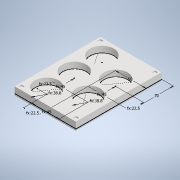
# Autodesk Inventor part: trayB
Saved by Autodesk Inventor 2022 (Build 260153000, 153)
## iProperties
Created: 2023-05-08
Part Number: trayB
Material: Generic
Document SubType Name: Modeling
Designer: Hallgato
Density: 1 g/cm^3
Appearance: Default
Author: Hallgato
Autodesk Inventor part; units mm, degrees
ref_plane "YZ Plane" through (0, 0, 0) normal (1, 0, 0) x (0, 1, 0)
ref_plane "XZ Plane" through (0, 0, 0) normal (0, 1, 0) x (-1, 0, 0)
ref_plane "XY Plane" through (0, 0, 0) normal (0, 0, 1) x (1, 0, 0)
sketch "Sketch1" plane through (0, 0, 0) normal (0, 1, 0) x (-1, 0, 0)
  circle A0 centre (0, 0) radius 19.4
  line L0 (0, 0) -> (0, -10.9961) construction
  circle A1 centre (0, -45) radius 19.4
  circle A2 centre (45, 22.5) radius 19.4
  circle A3 centre (45, -22.5) radius 19.4
  circle A4 centre (45, -67.5) radius 19.4
  line L1 (-27.5, -92.5) -> (72.5, -92.5)
  line L2 (72.5, -92.5) -> (72.5, 47.5)
  line L3 (72.5, 47.5) -> (-27.5, 47.5)
  line L4 (-27.5, 47.5) -> (-27.5, -92.5)
  line L5 (-27.5, -92.5) -> (72.5, 47.5) construction
  line L6 (72.5, -92.5) -> (-27.5, 47.5) construction
  point P0 (22.5, -22.5)
  dimension "d0" = 38.8
  dimension "d3" = 45
  dimension "d8" = 38.8
  dimension "d9" = 45
  dimension "d10" = 22.5
  dimension "d13" = 45
  dimension "d18" = 22.5
  dimension "d19" = 50
  dimension "d20" = 70
  dimension "d21" = 22.5
  constraints: 14 end point, 5 centre point, 3 vertical, 2 midpoint, 2 parallel, 1 coincident, 1 horizontal, 1 perpendicular, 6 other
  measures "d0" diameter of A0
  measures "d3" distance of L0.start A1.centre
  measures "d8" diameter of A2
  measures "d9" horizontal distance of A2.centre point (0, 0)
  measures "d10" vertical distance of point (0, 0) A2.centre
  measures "d13" distance of A2.centre A3.centre
  measures "d18" distance of point (22.5, -22.5) A3.centre
  measures "d19" distance from line of L4 point (22.5, -22.5)
  measures "d20" distance from line of L1 point (22.5, -22.5)
  measures "d21" horizontal distance of point (22.5, -22.5) A1.centre
extrude "Extrusion1" add sketch "Sketch1" along normal blind 10
extrude "Extrusion2" add sketch "Sketch1" against normal blind 3 contours A0 | A1 | A2 | A3 | A4 | L4 L3 L2 L1
sketch "Sketch3" plane through (0, 10, 0) normal (0, 1, 0) x (1, 0, 0)
  line L0 (24.5, 89.5) -> (19.5, 89.5)
  line L1 (19.5, 89.5) -> (19.5, 84.5)
  line L2 (19.5, 84.5) -> (24.5, 84.5)
  line L3 (24.5, 84.5) -> (24.5, 89.5)
  line L4 (24.5, -39.5) -> (19.5, -39.5)
  line L5 (19.5, -39.5) -> (19.5, -44.5)
  line L6 (19.5, -44.5) -> (24.5, -44.5)
  line L7 (24.5, -44.5) -> (24.5, -39.5)
  line L8 (-64.5, -44.5) -> (-69.5, -44.5)
  line L9 (-69.5, -44.5) -> (-69.5, -39.5)
  line L10 (-69.5, -39.5) -> (-64.5, -39.5)
  line L11 (-64.5, -39.5) -> (-64.5, -44.5)
  line L12 (-64.5, 89.5) -> (-69.5, 89.5)
  line L13 (-69.5, 89.5) -> (-69.5, 84.5)
  line L14 (-69.5, 84.5) -> (-64.5, 84.5)
  line L15 (-64.5, 84.5) -> (-64.5, 89.5)
  line L16 (27.5, -47.5) -> (27.5, 92.5) projected
  line L17 (27.5, 92.5) -> (-72.5, 92.5) projected
  line L18 (-72.5, -47.5) -> (27.5, -47.5) projected
  line L19 (-72.5, 92.5) -> (-72.5, -47.5) projected
  point P0 (0, 0)
  dimension "d26" = 5
  dimension "d27" = 3
  dimension "d28" = 3
  dimension "d29" = 5
  dimension "d30" = 3
  dimension "d31" = 3
  dimension "d32" = 5
  dimension "d33" = 3
  dimension "d34" = 5
  constraints: 32 end point, 8 parallel, 5 point on line, 4 horizontal, 4 perpendicular, 2 collinear
  measures "d26" distance between parallel lines of L2 L0
  measures "d27" distance between parallel lines of L16 L3
  measures "d28" distance between parallel lines of L17 L0
  measures "d29" distance between parallel lines of L3 L1
  measures "d30" distance between parallel lines of L18 L6
  measures "d31" distance between parallel lines of L16 L7
  measures "d32" distance between parallel lines of L6 L4
  measures "d33" distance between parallel lines of L13 L19
  measures "d34" distance between parallel lines of L11 L9
extrude "Extrusion3" cut sketch "Sketch3" against normal blind 2 contours L3 L2 L1 L0 | L7 L6 L5 L4 | L8 L9 L10 L11 | L15 L14 L13 L12
equation "\"d0\" = bottleDiameter"
equation "\"d3\" = bottleDistance"
equation "\"d8\" = bottleDiameter"
equation "\"d9\" = bottleDistance"
equation "\"d10\" = 0.5 * bottleDistance"
equation "\"d13\" = bottleDistance"
equation "\"d18\" = 0.5 * bottleDistance"
equation "\"d21\" = 0.5 * bottleDistance"
equation "\"capDiameter\" = 29.5"
equation "\"bottleLen\" = 81.3"
equation "\"bottleDiameter\" = 38.8"
equation "\"tubeInsideDiameter\" = 2"
equation "\"tubeOutsideDiameter\" = 5.4"
equation "\"tick\" = 2"
equation "\"connectorDiameter\" = 35"
equation "\"connectorInsideDiameter\" = tubeInsideDiameter - tick"
equation "\"connectorTubeDepth\" = 18.5"
equation "\"tubeFlapDepth\" = 3"
equation "\"tubeFlapAngle\" = 15deg"
equation "\"minTick\" = 0.25"
equation "\"tubeLinkTick\" = 2"
equation "\"tubeTolerance\" = 0.3"
equation "\"tickHolder\" = 1"
equation "\"bottleDistance\" = 45"
body "Solid1"
